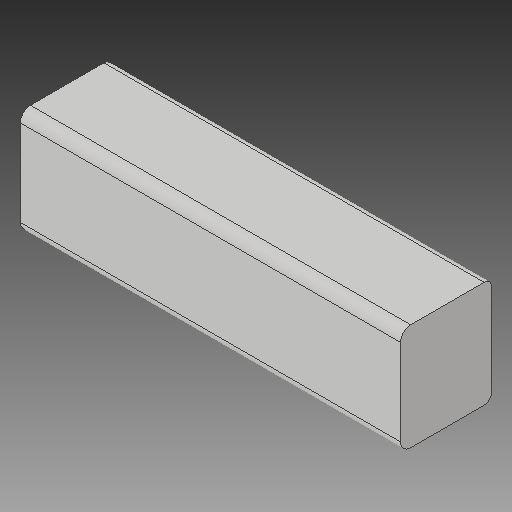
# Autodesk Inventor part: Batt
Saved by Autodesk Inventor 2019 (Build 230136000, 136)
## iProperties
Created: 2020-02-04
Part Number: Batt
Material: Generic
Document SubType Name: Modeling
Designer: peter
Density: 1 g/cm^3
Appearance: Default
Mass: 28.1488 g
Surface Area: 63.753 cm^2
Volume: 28.1488 cm^3
Author: peter
Autodesk Inventor part; units mm, degrees
ref_plane "YZ Plane" through (0, 0, 0) normal (1, 0, 0) x (0, 1, 0)
ref_plane "XZ Plane" through (0, 0, 0) normal (0, 1, 0) x (-1, 0, 0)
ref_plane "XY Plane" through (0, 0, 0) normal (0, 0, 1) x (1, 0, 0)
sketch "Sketch1" plane through (0, 0, 0) normal (1, 0, 0) x (0, 1, 0)
  line L0 (11.8859, -6.6669) -> (-5.1141, -6.6669)
  line L1 (-7.1141, -8.6669) -> (-7.1141, -23.1669)
  line L2 (-5.6141, -24.6669) -> (12.3859, -24.6669)
  line L3 (13.8859, -23.1669) -> (13.8859, -8.6669)
  arc A0 (13.8859, -8.6669) -> (11.8859, -6.6669) centre (11.8859, -8.6669) ccw
  arc A1 (-5.1141, -6.6669) -> (-7.1141, -8.6669) centre (-5.1141, -8.6669) ccw
  arc A2 (12.3859, -24.6669) -> (13.8859, -23.1669) centre (12.3859, -23.1669) ccw
  arc A3 (-7.1141, -23.1669) -> (-5.6141, -24.6669) centre (-5.6141, -23.1669) ccw
  point P0 (0, 0)
  point P1 (-7.1141, -24.6669)
  point P2 (-7.1141, -6.6669)
  point P3 (13.8859, -24.6669)
  dimension "d0" = 21
  dimension "d1" = 18
  dimension "d2" = 2
  dimension "d3" = 1.5
  constraints: 8 end point, 8 point on circle, 8 tangent, 6 point on line, 4 centre point, 2 equal radius, 2 parallel, 1 horizontal, 1 perpendicular
  measures "d0" distance of point (13.886, -24.667) point (-7.114, -24.667)
  measures "d1" distance of point (-7.114, -24.667) point (-7.114, -6.667)
  measures "d2" radius of A0
  measures "d3" radius of A2
extrude "Extrusion1" add sketch "Sketch1" along normal blind 75
body "Solid1"
